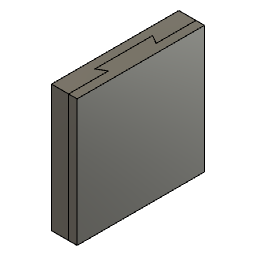
tool-connector (Autodesk Fusion 360 design; units mm, degrees)
Autodesk Fusion 360 part; units mm, degrees
sketch "Sketch2" plane through (0, 0, 0) normal (1, 0, 0) x (0, 0, -1)
  line L0 (-37.3127, 37.1798) -> (37.3127, 37.1798)
  line L1 (37.3127, 37.1798) -> (37.3127, -37.1798)
  line L2 (37.3127, -37.1798) -> (-37.3127, -37.1798)
  line L3 (-37.3127, -37.1798) -> (-37.3127, 37.1798)
  line L4 (0, 62.0565) -> (0, -42.698) construction
  line L5 (-61.9952, 0) -> (63.5549, 0) construction
  line L6 (-24.4856, -37.1798) -> (-13.9907, 37.1798)
  line L7 (13.9907, 37.1798) -> (24.4856, -37.1798)
  constraint horizontal L0
  constraint vertical L1
  constraint horizontal L2
  constraint vertical L3
  constraint vertical L4
  constraint horizontal L5
  constraint coincident origin L4
  constraint coincident origin L5
  constraint symmetric L1 L3 L4
  constraint symmetric L0 L2 L5
  constraint coincident L2 L6.start
  constraint coincident L0 L6.end
  constraint coincident L0 L7.start
  constraint coincident L2 L7.end
  constraint symmetric L4 L6.end L7.start
  constraint symmetric L4 L6.start L7.end
extrude "Extrude1" add sketch "Sketch2" along normal blind 10 contours L0 L2 L3 L6 | L0 L1 L2 L7 makes body 1 at (0, 12.3933, 25.263) makes body 2 at (0, 12.3933, -25.263)
extrude "Extrude2" add sketch "Sketch2" along normal blind 5 contours L0 L2 L6 L7 bodies 1 2
draft "Draft1" angle -30 neutral plane through (10, 0, 0) pull (1, 0, 0) 1 faces at (8.3333, -12.3933, 20.9873) on bodies 1
draft "Draft2" angle -30 neutral plane through (10, 0, 0) pull (1, 0, 0) 1 faces at (8.3333, 12.3933, -17.489) on bodies 1
sketch "Sketch3" plane through (5, 0, 0) normal (1, 0, 0) x (0, 0, -1)
  line L0 (16.9061, 37.1798) -> (-16.9061, 37.1798)
  line L1 (-16.9061, 37.1798) -> (-27.401, -37.1798)
  line L2 (-27.401, -37.1798) -> (27.401, -37.1798)
  line L3 (27.401, -37.1798) -> (16.9061, 37.1798)
  circle A0 centre (0, -18.4044) radius 4
  line L4 (0, 0) -> (0, -18.4044) construction
  dimension "d9" = 8
  constraint coincident L4.start origin
  constraint coincident A0.centre L4.end
  constraint vertical L4
  measures "d9" diameter of A0
extrude "Extrude3" cut sketch "Sketch3" against normal blind 3 contours A0 bodies 1
copy_body "Body->Comp1" bodies 1 removing the originals makes body 3 in component "base"
copy_body "CopyPasteBodies1" bodies 3 makes body 4
sketch "Sketch4" plane through (5, 0, 0) normal (1, 0, 0) x (0, 0, -1)
  circle A0 centre (0, -18.4044) radius 4
  line L0 (16.9061, 37.1798) -> (-16.9061, 37.1798)
  line L1 (-16.9061, 37.1798) -> (-27.401, -37.1798) construction
  line L2 (-27.401, -37.1798) -> (27.401, -37.1798)
  line L3 (27.401, -37.1798) -> (16.9061, 37.1798) construction
  line L4 (-37.3127, 37.1798) -> (37.3127, 37.1798)
  line L5 (37.3127, 37.1798) -> (37.3127, -37.1798)
  line L6 (37.3127, -37.1798) -> (-37.3127, -37.1798)
  line L7 (-37.3127, -37.1798) -> (-37.3127, 37.1798)
  point P0 (-37.3127, 37.1798)
  point P1 (37.3127, -37.1798)
  constraint horizontal L4
  constraint vertical L5
  constraint horizontal L6
  constraint vertical L7
  constraint coincident P1 L5.end
  constraint coincident P0 L4.start
extrude "Extrude4" add sketch "Sketch4" along normal blind 10 separate body makes body 5
combine "Combine1" operation cut target body 5 tool bodies 4
delete_face "DeleteFace1" 1 faces at (11.6667, -18.6038, -3.995) on bodies 5
extrude "Extrude5" cut sketch "Sketch3" along normal blind 3 contours A0 bodies 5
copy_body "Body->Comp2" bodies 5 removing the originals makes body 6 in component "tool_plate"
component "base" placed x (1, 0, 0) y (0, 1, 0) z (0, 0, 1) at (0, 0, 0)
component "tool_plate" placed x (1, 0, 0) y (0, 1, 0) z (0, 0, 1) at (0, 0, 0)
named bodies: "base", "tool_plate"
